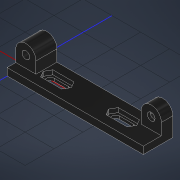
# Autodesk Inventor part: Door_Panel
Saved by Autodesk Inventor 2022.2 (Build 262287010, 287A)
## iProperties
Created: 2022-01-24
Part Number: Door_Panel
Material: ABS-Kunststoff
Document SubType Name: Modeling
Designer: sleib
Density: 1.06 g/cm^3
Appearance: Glatt - Schwarz
Author: sleib
Autodesk Inventor part; units mm, degrees
ref_plane "YZ Plane" through (0, 0, 0) normal (1, 0, 0) x (0, 1, 0)
ref_plane "XZ Plane" through (0, 0, 0) normal (0, 1, 0) x (-1, 0, 0)
ref_plane "XY Plane" through (0, 0, 0) normal (0, 0, 1) x (1, 0, 0)
sketch "Skizze1" plane through (0, 0, 0) normal (0, 0, 1) x (1, 0, 0)
  circle A0 centre (7, 13) radius 2.65
  circle A1 centre (87.334, 13) radius 2.65
  arc A2 (14, 13) -> (0, 13) centre (7, 13) ccw
  arc A3 (94.334, 13) -> (80.334, 13) centre (87.334, 13) ccw
  line L0 (94.334, 0) -> (0, 0)
  line L1 (0, 5) -> (94.334, 5)
  line L2 (94.334, 13) -> (94.334, 0)
  line L3 (80.334, 13) -> (80.334, 5)
  line L4 (14, 13) -> (14, 5)
  line L5 (0, 13) -> (0, 0)
  dimension "d4" = 5.3
  dimension "d5" = 5.3
  dimension "d8" = 80.334
  dimension "d18" = 5
  dimension "d21" = 7
  dimension "d22" = 13
  constraints: 12 end point, 4 centre point, 4 point on circle, 4 point on line, 4 tangent, 2 concentric, 2 perpendicular, 2 vertical, 1 coincident, 1 equal radius, 1 horizontal, 1 horizontal alignment, 1 parallel
  measures "d4" diameter of A0
  measures "d5" diameter of A1
  measures "d8" distance of A1.centre A0.centre
  measures "d18" distance between parallel lines of L1 L0
  measures "d21" radius of A3
  measures "d22" distance from line of A1.centre L0
extrude "Extrusion1" add sketch "Skizze1" along normal blind 12.5 and the other way blind 8 contours L1 L2 L0 L5
extrude "Extrusion2" add sketch "Skizze1" against normal blind 8 contours L3 A3 L2 L1
extrude "Extrusion3" add sketch "Skizze1" along normal blind 6.5 and the other way blind 8 contours L4 L1 L5 A2
sketch "Skizze2" plane through (0, 0, -8) normal (0, 0, -1) x (-1, 0, 0)
  circle A0 centre (-87.334, 13) radius 2.65 projected
  circle A1 centre (-7, 13) radius 2.65 projected
  line L0 (-87.334, 17.9075) -> (-83.084, 15.4537)
  line L1 (-83.084, 15.4537) -> (-83.084, 10.5463)
  line L2 (-83.084, 10.5463) -> (-87.334, 8.0925)
  line L3 (-87.334, 8.0925) -> (-91.584, 10.5463)
  line L4 (-91.584, 10.5463) -> (-91.584, 15.4537)
  line L5 (-91.584, 15.4537) -> (-87.334, 17.9075)
  line L6 (-7, 17.9075) -> (-2.75, 15.4537)
  line L7 (-2.75, 15.4537) -> (-2.75, 10.5463)
  line L8 (-2.75, 10.5463) -> (-7, 8.0925)
  line L9 (-7, 8.0925) -> (-11.25, 10.5463)
  line L10 (-11.25, 10.5463) -> (-11.25, 15.4537)
  line L11 (-11.25, 15.4537) -> (-7, 17.9075)
  point P0 (0, 0)
  dimension "d23" = 8.5
  dimension "d24" = 8.5
  constraints: 24 end point, 2 coincident, 2 vertical, 26 other
  measures "d23" distance between parallel lines of L1 L4
  measures "d24" distance between parallel lines of L7 L10
extrude "Extrusion4" cut sketch "Skizze2" against normal blind 6 contours L0 L1 L2 L3 L4 L5
extrude "Extrusion5" cut sketch "Skizze2" against normal blind 6 contours A1 | L6 L7 L8 L9 L10 L11
sketch "Skizze3" plane through (0, 0, 12.5) normal (0, -1, 0) x (1, 0, 0)
  line L0 (94.334, 0) -> (94.334, -20.5) projected
  line L1 (0, 0) -> (94.334, 0) projected
  line L2 (0, -20.5) -> (0, 0) projected
  line L3 (94.334, -20.5) -> (0, -20.5) projected
  line L4 (0, -20.5) -> (0, 0) projected
  line L5 (0, -10.25) -> (94.334, -10.25) construction
  line L6 (94.334, 0) -> (94.334, -20.5) projected
  line L7 (17, -10.25) -> (32, -10.25) construction
  line L8 (19.65, -12.9) -> (29.35, -12.9)
  line L9 (29.35, -7.6) -> (19.65, -7.6)
  arc A0 (19.65, -7.6) -> (19.65, -12.9) centre (19.65, -10.25) ccw
  arc A1 (29.35, -12.9) -> (29.35, -7.6) centre (29.35, -10.25) ccw
  line L10 (62.334, -10.25) -> (77.334, -10.25) construction
  line L11 (64.984, -12.9) -> (74.684, -12.9)
  line L12 (74.684, -7.6) -> (64.984, -7.6)
  arc A2 (64.984, -7.6) -> (64.984, -12.9) centre (64.984, -10.25) ccw
  arc A3 (74.684, -12.9) -> (74.684, -7.6) centre (74.684, -10.25) ccw
  point P0 (0, -12.5)
  point P1 (24.5, -10.25)
  point P2 (69.834, -10.25)
  dimension "d34" = 5.3
  dimension "d35" = 5.3
  dimension "d36" = 15
  dimension "d37" = 15
  dimension "d38" = 17
  dimension "d39" = 17
  constraints: 18 end point, 12 point on circle, 8 point on line, 8 tangent, 4 centre point, 4 midpoint, 2 parallel
  measures "d34" distance between parallel lines of L8 L9
  measures "d35" distance between parallel lines of L11 L12
  measures "d36" distance of L7.end L7.start
  measures "d37" distance of L10.end L10.start
  measures "d38" distance from line of L7.start L2
  measures "d39" distance from line of L0 L10.end
extrude "Extrusion6" cut sketch "Skizze3" against normal through all contours A0 L9 A1 L8 | A2 L12 A3 L11
sketch "Skizze4" plane through (0, 5, 12.5) normal (0, 1, 0) x (1, 0, 0)
  line L0 (74.684, 7.6) -> (64.984, 7.6) projected
  arc A0 (64.984, 12.9) -> (64.984, 7.6) centre (64.984, 10.25) ccw projected
  line L1 (64.984, 12.9) -> (74.684, 12.9) projected
  arc A1 (74.684, 7.6) -> (74.684, 12.9) centre (74.684, 10.25) ccw projected
  line L2 (29.35, 7.6) -> (19.65, 7.6) projected
  arc A2 (19.65, 12.9) -> (19.65, 7.6) centre (19.65, 10.25) ccw projected
  line L3 (19.65, 12.9) -> (29.35, 12.9) projected
  arc A3 (29.35, 7.6) -> (29.35, 12.9) centre (29.35, 10.25) ccw projected
  line L4 (14, 6) -> (0, 6) projected
  line L5 (0, 6) -> (0, 0) projected
  line L6 (94.334, 0) -> (0, 0) projected
  line L7 (94.334, 12.5) -> (94.334, 0) projected
  line L8 (94.334, 12.5) -> (80.334, 12.5) projected
  line L9 (80.334, 12.5) -> (80.334, 20.5) projected
  line L10 (14, 20.5) -> (80.334, 20.5) projected
  line L11 (14, 20.5) -> (14, 6) projected
  line L12 (77.1378, 6) -> (72.2303, 6)
  line L13 (72.2303, 6) -> (69.7765, 10.25)
  line L14 (69.7765, 10.25) -> (72.2303, 14.5)
  line L15 (72.2303, 14.5) -> (77.1378, 14.5)
  line L16 (77.1378, 14.5) -> (79.5915, 10.25)
  line L17 (79.5915, 10.25) -> (77.1378, 6)
  line L18 (62.5303, 6) -> (60.0765, 10.25)
  line L19 (60.0765, 10.25) -> (62.5303, 14.5)
  line L20 (62.5303, 14.5) -> (67.4378, 14.5)
  line L21 (67.4378, 14.5) -> (69.8915, 10.25)
  line L22 (69.8915, 10.25) -> (67.4378, 6)
  line L23 (67.4378, 6) -> (62.5303, 6)
  line L24 (31.8037, 6) -> (26.8963, 6)
  line L25 (26.8963, 6) -> (24.4425, 10.25)
  line L26 (24.4425, 10.25) -> (26.8963, 14.5)
  line L27 (26.8963, 14.5) -> (31.8037, 14.5)
  line L28 (31.8037, 14.5) -> (34.2575, 10.25)
  line L29 (34.2575, 10.25) -> (31.8037, 6)
  line L30 (17.1963, 6) -> (14.7425, 10.25)
  line L31 (14.7425, 10.25) -> (17.1963, 14.5)
  line L32 (17.1963, 14.5) -> (22.1037, 14.5)
  line L33 (22.1037, 14.5) -> (24.5575, 10.25)
  line L34 (24.5575, 10.25) -> (22.1037, 6)
  line L35 (22.1037, 6) -> (17.1963, 6)
  line L36 (72.2303, 6) -> (67.4378, 6)
  line L37 (74.684, 7.6) -> (64.984, 7.6) projected
  line L38 (72.2303, 14.5) -> (67.4378, 14.5)
  line L39 (26.8963, 6) -> (22.1037, 6)
  line L40 (26.8963, 14.5) -> (22.1037, 14.5)
  point P0 (0, 12.5)
  dimension "d42" = 8.5
  constraints: 56 end point, 4 coincident, 4 horizontal, 4 parallel, 3 collinear, 52 other
  measures "d42" distance between parallel lines of L15 L12
extrude "Extrusion7" cut sketch "Skizze4" against normal blind 3 contours A1 L1 L14 L15 L16 L17 L12 L13 L0 | L13 L36 L22 L0 | L22 L23 L18 L19 L20 L21 L1 A0 L0 | L1 L21 L38 L14 | A3 L3 L26 L27 L28 L29 L24 L25 L2 | L25 L39 L34 L2 | L34 L35 L30 L31 L32 L33 L3 A2 L2 | L3 L33 L40 L26
equation "\"d4\" = d5"
equation "\"d10\" = d14"
equation "\"d29\" = d14"
equation "\"d24\" = d23"
equation "\"d35\" = d34"
equation "\"d37\" = d36"
equation "\"d14\" = 8"
